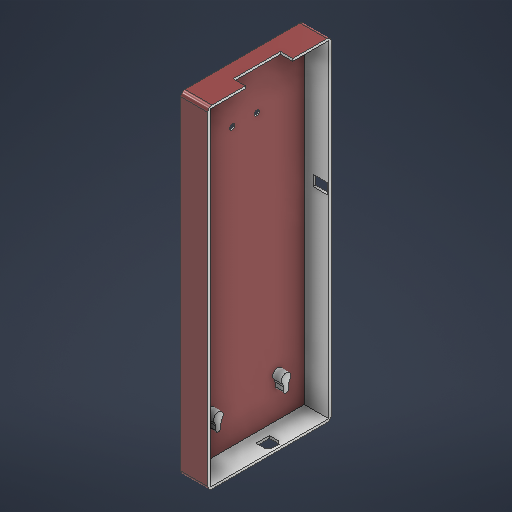
# Autodesk Inventor part: cDAQ_Bottom_Box3
Saved by Autodesk Inventor 2027 (Build 310192000, 192)
## iProperties
Created: 2026-05-08
Part Number: cDAQ_Bottom_Box3
Material: Generic
Document SubType Name: Modeling
Designer: giese
Density: 1 g/cm^3
Appearance: Default
Author: giese
Autodesk Inventor part; units mm, degrees
ref_plane "YZ Plane" through (0, 0, 0) normal (1, 0, 0) x (0, 1, 0)
ref_plane "XZ Plane" through (0, 0, 0) normal (0, 1, 0) x (-1, 0, 0)
ref_plane "XY Plane" through (0, 0, 0) normal (0, 0, 1) x (1, 0, 0)
sketch "Sketch1" plane through (0, 0, 0) normal (1, 0, 0) x (0, 1, 0)
  line L0 (37.5698, 44.2767) -> (-211.9852, 44.2767)
  line L1 (-211.9852, 44.2767) -> (-211.9852, -48.4333)
  line L2 (-211.9852, -48.4333) -> (37.5698, -48.4333)
  line L3 (37.5698, -48.4333) -> (37.5698, 44.2767)
  point P0 (0, 0)
  dimension "d0" = 92.71
  dimension "d1" = 249.555
  constraints: 8 end point, 2 parallel, 1 horizontal, 1 perpendicular
  measures "d0" distance of L2.end L0.start
  measures "d1" distance of L1.end L2.end
extrude "Extrusion1" add sketch "Sketch1" along normal blind 20.32
sketch "Sketch2" plane through (20.32, 0, 0) normal (1, 0, 0) x (0, 0, -1)
  line L0 (46.5283, 35.6648) -> (-42.3717, 35.6648)
  line L1 (-42.3717, 35.6648) -> (-42.3717, -210.0802)
  line L2 (-42.3717, -210.0802) -> (46.5283, -210.0802)
  line L3 (46.5283, -210.0802) -> (46.5283, 35.6648)
  line L4 (48.4333, 37.5698) -> (-44.2767, 37.5698) projected
  line L5 (-44.2767, 37.5698) -> (-44.2767, -211.9852) projected
  point P0 (0, 0)
  dimension "d4" = 245.745
  dimension "d5" = 88.9
  dimension "d8" = 1.905
  dimension "d21" = 1.905
  constraints: 8 end point, 2 parallel, 1 horizontal, 1 perpendicular
  measures "d4" distance of L2.end L0.start
  measures "d5" distance of L0.start L0.end
  measures "d8" distance between parallel lines of L0 L4
  measures "d21" distance between parallel lines of L5 L1
extrude "Extrusion2" cut sketch "Sketch2" against normal blind 18.415
sketch "Sketch3" plane through (0, 0, 0) normal (-1, 0, 0) x (0, 0, 1)
  circle A0 centre (-11.0089, -2.6638) radius 2
  circle A1 centre (7.4899, -2.6638) radius 2
  circle A2 centre (25.9887, -2.6638) radius 2
  line L0 (-48.4333, -211.9852) -> (-48.4333, 37.5698) projected
  line L1 (-48.4333, 37.5698) -> (44.2767, 37.5698) projected
  line L2 (44.2767, 37.5698) -> (44.2767, -211.9852) projected
  line L3 (42.3717, 35.6648) -> (-46.5283, 35.6648) projected
  point P0 (0, 0)
  point P1 (-0.896, -23.7433)
  point P2 (-45.1848, 27.0137)
  dimension "d9" = 18.4988
  dimension "d10" = 4
  dimension "d11" = 4
  dimension "d12" = 18.4988
  dimension "d13" = 36.9976
  dimension "d18" = 18.288
  dimension "d22" = 4
  dimension "d58" = 40.2336
  constraints: 3 centre point
  measures "d9" distance of A0.centre A1.centre
  measures "d10" diameter of A1
  measures "d11" diameter of A2
  measures "d12" distance of A1.centre A2.centre
  measures "d13" distance of A0.centre A2.centre
  measures "d18" distance from line of L2 A2.centre
  measures "d22" diameter of A0
  measures "d58" distance from line of L1 A2.centre
extrude "Extrusion3" cut sketch "Sketch3" against normal blind 3.81
sketch "Sketch5" plane through (0, -211.9852, -48.4333) normal (0, 0, -1) x (-1, 0, 0)
  line L0 (-19.2532, 146.8628) -> (-8.5598, 146.8628)
  line L1 (-8.5598, 146.8628) -> (-8.5598, 154.8628)
  line L2 (-8.5598, 154.8628) -> (-19.2532, 154.8628)
  line L3 (-19.2532, 154.8628) -> (-19.2532, 146.8628)
  line L4 (0, 249.555) -> (-20.32, 249.555) projected
  line L5 (0, 0) -> (0, 249.555) projected
  point P0 (0, 211.9852)
  point P1 (-13.9065, 154.8628)
  point P2 (-13.9065, 146.8628)
  dimension "d28" = 10.6934
  dimension "d30" = 8
  dimension "d31" = 8.5598
  dimension "d34" = 102.6922
  constraints: 8 end point, 2 midpoint, 2 parallel, 1 horizontal, 1 perpendicular
  measures "d28" distance between parallel lines of L1 L3
  measures "d30" distance of point (-13.907, 154.863) point (-13.907, 146.863)
  measures "d31" distance between parallel lines of L5 L1
  measures "d34" distance between parallel lines of L4 L0
extrude "Extrusion4" cut sketch "Sketch5" against normal blind 24.13
sketch "Sketch6" plane through (0, -211.9852, -48.4333) normal (0, -1, 0) x (1, 0, 0)
  line L0 (16, 45.1284) -> (9, 45.1284)
  line L1 (9, 45.1284) -> (9, 35.1284)
  line L2 (9, 35.1284) -> (16, 35.1284)
  line L3 (0, 92.71) -> (0, 0) projected
  line L4 (18.24, 43.1283) -> (18.24, 37.1284)
  line L5 (16, 45.1284) -> (18.24, 43.1283)
  line L6 (18.24, 37.1284) -> (16, 35.1284)
  line L7 (0, 0) -> (20.32, 0) projected
  point P0 (0, 48.4333)
  point P1 (12.5, 45.1284)
  point P2 (12.5, 35.1284)
  dimension "d35" = 10
  dimension "d39" = 6
  dimension "d48" = 45.1284
  dimension "d49" = 18.24
  constraints: 12 end point, 2 midpoint, 1 horizontal, 1 parallel, 1 perpendicular, 1 vertical
  measures "d35" distance of point (12.5, 45.128) point (12.5, 35.128)
  measures "d39" distance of L4.start L4.end
  measures "d48" distance between parallel lines of L7 L0
  measures "d49" distance between parallel lines of L3 L4
extrude "Extrusion5" cut sketch "Sketch6" against normal blind 3.81
sketch "Sketch7" plane through (0, 37.5698, 44.2767) normal (0, 1, 0) x (1, 0, 0)
  line L0 (26.1366, 63.754) -> (11.1252, 63.754)
  line L1 (11.1252, 63.754) -> (11.1252, 28.194)
  line L2 (11.1252, 28.194) -> (26.1366, 28.194)
  line L3 (26.1366, 28.194) -> (26.1366, 63.754)
  line L4 (0, 0) -> (20.32, 0) projected
  line L5 (0, 92.71) -> (0, 0) projected
  line L6 (20.32, 92.71) -> (20.32, 0) projected
  point P0 (0, 44.2767)
  dimension "d51" = 35.56
  dimension "d52" = 28.194
  dimension "d55" = 11.1252
  dimension "d56" = 15.0114
  dimension "d57" = 5.8166
  constraints: 8 end point, 2 parallel, 1 horizontal, 1 perpendicular
  measures "d51" distance of L2.end L0.start
  measures "d52" distance between parallel lines of L4 L2
  measures "d55" distance between parallel lines of L5 L1
  measures "d56" distance between parallel lines of L3 L1
  measures "d57" distance between parallel lines of L6 L3
extrude "Extrusion6" cut sketch "Sketch7" against normal blind 3.81
fillet "Fillet1" radius 3.175 4 edges at (10.16, 37.5698, -48.4333) (10.16, 37.5698, 44.2767) (10.16, -211.9852, -48.4333) (10.16, -211.9852, 44.2767)
sketch "Sketch8" plane through (0, 0, 0) normal (-1, 0, 0) x (0, 0, 1)
  line L0 (-12.7805, -6.1944) -> (-9.2499, -6.1944)
  line L1 (-12.7805, 0.8668) -> (-9.2499, 0.8668)
  line L2 (-12.7805, -6.1944) -> (-14.8189, -2.6638)
  line L3 (-12.7805, 0.8668) -> (-14.8189, -2.6638)
  line L4 (-9.2499, -6.1944) -> (-7.2116, -2.6638)
  line L5 (-9.2499, 0.8668) -> (-7.2116, -2.6638)
  circle A0 centre (-11.0089, -2.6638) radius 2 projected
  line L6 (5.7183, -6.1944) -> (9.2489, -6.1944)
  line L7 (5.7183, 0.8668) -> (9.2489, 0.8668)
  line L8 (5.7183, -6.1944) -> (3.6799, -2.6638)
  line L9 (5.7183, 0.8668) -> (3.6799, -2.6638)
  line L10 (9.2489, -6.1944) -> (11.2873, -2.6638)
  line L11 (9.2489, 0.8668) -> (11.2873, -2.6638)
  circle A1 centre (7.4899, -2.6638) radius 2 projected
  line L12 (24.2171, -6.1944) -> (22.1787, -2.6638)
  line L13 (24.2171, 0.8668) -> (22.1787, -2.6638)
  line L14 (24.2171, -6.1944) -> (27.7477, -6.1944)
  line L15 (24.2171, 0.8668) -> (27.7477, 0.8668)
  line L16 (27.7477, -6.1944) -> (29.7861, -2.6638)
  line L17 (27.7477, 0.8668) -> (29.7861, -2.6638)
  circle A2 centre (25.9887, -2.6638) radius 2 projected
  point P0 (-11.0152, -6.1944)
  point P1 (7.4836, -6.1944)
  point P2 (25.9824, -6.1944)
  dimension "d60" = 7.0612
  dimension "d61" = 120
  dimension "d62" = 120
  dimension "d63" = 120
  dimension "d64" = 120
  dimension "d65" = 3.5306
  dimension "d66" = 3.5306
  dimension "d67" = 3.5306
  dimension "d68" = 3.5306
  dimension "d69" = 3.5306
  dimension "d70" = 3.5306
  dimension "d71" = 0
  dimension "d72" = 7.6074
  dimension "d73" = 3.81
  dimension "d74" = 0
  dimension "d75" = 7.0612
  dimension "d76" = 120
  dimension "d77" = 120
  dimension "d78" = 120
  dimension "d79" = 120
  dimension "d80" = 3.5306
  dimension "d81" = 3.5306
  dimension "d82" = 3.5306
  dimension "d83" = 3.5306
  dimension "d84" = 3.5306
  dimension "d85" = 3.5306
  dimension "d86" = 0
  dimension "d87" = 7.6074
  dimension "d91" = 0
  dimension "d92" = 3.81
  dimension "d93" = 7.0612
  dimension "d94" = 120
  dimension "d95" = 120
  dimension "d96" = 120
  dimension "d97" = 120
  dimension "d98" = 3.5306
  dimension "d99" = 3.5306
  dimension "d100" = 3.5306
  dimension "d101" = 3.5306
  dimension "d102" = 3.5306
  dimension "d103" = 3.5306
  dimension "d104" = 0
  dimension "d105" = 7.6074
  dimension "d108" = 0
  dimension "d109" = 3.81
  constraints: 36 end point, 6 horizontal, 3 midpoint
  measures "d60" distance from line of point (-11.015, -6.194) L1
  measures "d61" angle of L0 L2
  measures "d62" angle of L1 L3
  measures "d63" angle of L4 L0
  measures "d64" angle of L5 L1
  measures "d65" distance of L0.start L0.end
  measures "d66" distance of L1.start L1.end
  measures "d67" vertical distance of L1.start L3.end
  measures "d68" vertical distance of L0.start L2.end
  measures "d69" vertical distance of L1.end L5.end
  measures "d70" vertical distance of L0.end L4.end
  measures "d71" horizontal distance of L0.start L1.start
  measures "d72" distance of L4.end L2.end
  measures "d73" distance of A0.centre L2.end
  measures "d74" vertical distance of A0.centre L4.end
  measures "d75" distance from line of point (7.484, -6.194) L7
  measures "d76" angle of L6 L8
  measures "d77" angle of L7 L9
  measures "d78" angle of L10 L6
  measures "d79" angle of L11 L7
  measures "d80" distance of L8.start L6.end
  measures "d81" distance of L9.start L7.end
  measures "d82" vertical distance of L9.start L9.end
  measures "d83" vertical distance of L8.start L8.end
  measures "d84" vertical distance of L7.end L11.end
  measures "d85" vertical distance of L6.end L10.end
  measures "d86" horizontal distance of L8.start L9.start
  measures "d87" distance of L10.end L8.end
  measures "d91" vertical distance of A1.centre L8.end
  measures "d92" distance of A1.centre L8.end
  measures "d93" distance from line of point (25.982, -6.194) L15
  measures "d94" angle of L14 L12
  measures "d95" angle of L15 L13
  measures "d96" angle of L16 L14
  measures "d97" angle of L17 L15
  measures "d98" distance of L12.start L16.start
  measures "d99" distance of L15.start L15.end
  measures "d100" vertical distance of L15.start L13.end
  measures "d101" vertical distance of L12.start L12.end
  measures "d102" vertical distance of L15.end L17.end
  measures "d103" vertical distance of L16.start L16.end
  measures "d104" horizontal distance of L12.start L15.start
  measures "d105" distance of L16.end L12.end
  measures "d108" vertical distance of A2.centre L12.end
  measures "d109" distance of A2.centre L12.end
extrude "Extrusion7" cut sketch "Sketch8" against normal blind 0.9525 contours L2 L3 L1 L5 L4 L0 | A0 | L8 L9 L7 L11 L10 L6 | A1 | L12 L13 L15 L17 L16 L14 | A2
sketch "Sketch9" plane through (1.905, 0, 0) normal (1, 0, 0) x (0, 0, -1)
  arc A0 (29.2539, -182.3284) -> (23.7977, -182.3284) centre (26.5258, -179.8542) ccw
  line L0 (45.2583, 37.5698) -> (19.4773, 37.5698) projected
  line L1 (46.5283, 35.6648) -> (46.5283, -210.0802) projected
  arc A1 (24.6208, -187.4742) -> (28.4308, -187.4742) centre (26.5258, -187.4742) ccw
  line L2 (28.4308, -187.4742) -> (28.4308, -184.4614)
  line L3 (24.6208, -187.4742) -> (24.6208, -184.4614)
  arc A2 (29.2539, -182.3284) -> (28.4308, -184.4614) centre (31.6058, -184.4614) ccw
  arc A3 (24.6208, -184.4614) -> (23.7977, -182.3284) centre (21.4458, -184.4614) ccw
  arc A4 (-21.5461, -182.3284) -> (-27.0023, -182.3285) centre (-24.2742, -179.8542) ccw
  arc A5 (-26.1792, -187.4606) -> (-22.3692, -187.4742) centre (-24.2742, -187.4742) ccw
  line L4 (-22.3692, -187.4742) -> (-22.3692, -184.4614)
  line L5 (-26.1792, -187.4606) -> (-26.1792, -184.4614)
  arc A6 (-21.5461, -182.3284) -> (-22.3692, -184.4614) centre (-19.1942, -184.4614) ccw
  arc A7 (-26.1792, -184.4614) -> (-27.0023, -182.3285) centre (-29.3542, -184.4614) ccw
  line L6 (-16.0827, 37.5698) -> (-41.1017, 37.5698) projected
  line L7 (-42.3717, -210.0802) -> (-42.3717, 35.6648) projected
  point P0 (0, 0)
  point P1 (28.4308, -183.0063)
  point P2 (24.6208, -183.0063)
  point P3 (-22.3692, -183.0063)
  point P4 (-26.1792, -183.0063)
  dimension "d112" = 217.424
  dimension "d114" = 7.366
  dimension "d116" = 3.81
  dimension "d117" = 225.044
  dimension "d118" = 3.175
  dimension "d119" = 7.366
  dimension "d120" = 3.81
  dimension "d121" = 3.175
  dimension "d122" = 217.424
  dimension "d123" = 225.044
  dimension "d125" = 0
  dimension "d128" = 50.8
  dimension "d129" = 20.0025
  dimension "d130" = 0
  constraints: 20 point on circle, 8 centre point, 8 end point, 8 tangent, 4 point on line, 2 equal radius, 2 parallel, 2 vertical
  measures "d112" distance from line of L0 A0.centre
  measures "d114" diameter of A0
  measures "d116" diameter of A1
  measures "d117" distance from line of L0 A1.centre
  measures "d118" radius of A2
  measures "d119" diameter of A4
  measures "d120" diameter of A5
  measures "d121" radius of A6
  measures "d122" distance from line of A4.centre L6
  measures "d123" distance from line of L6 A5.centre
  measures "d125" horizontal distance of A5.centre A4.centre
  measures "d128" distance of A5.centre A1.centre
  measures "d129" distance from line of L1 A0.centre
  measures "d130" horizontal distance of A0.centre A1.centre
extrude "Extrusion8" add sketch "Sketch9" along normal blind 6.4008
body "Solid1"
